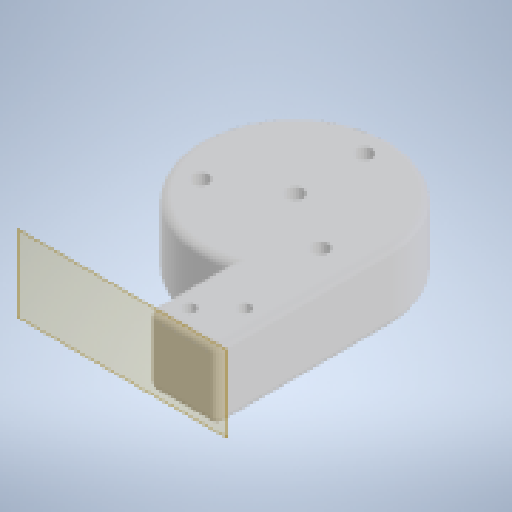
# Autodesk Inventor part: PulleytoHand
Saved by Autodesk Inventor 2024 (Build 280153000, 153)
## iProperties
Created: 2024-02-21
Part Number: PulleytoHand
Material: PC/ABS Plastic
Document SubType Name: Modeling
Designer: Irwin
Density: 0.357273 g/cm^3
Appearance: Smooth - White
Author: Irwin
Autodesk Inventor part; units mm, degrees
ref_plane "YZ Plane" through (0, 0, 0) normal (1, 0, 0) x (0, 1, 0)
ref_plane "XZ Plane" through (0, 0, 0) normal (0, 1, 0) x (-1, 0, 0)
sketch "Sketch1" plane through (0, 0, 0) normal (0, 1, 0) x (-1, 0, 0)
  circle A0 centre (0, 0) radius 27.5
  dimension "d0" = 55
  constraints: 1 centre point, 1 coincident
  measures "d0" diameter of A0
extrude "Extrusion1" add sketch "Sketch1" along normal blind 20
ref_plane "Work Plane1" through (0, 0, 50) normal (0, 0, 1) x (1, 0, 0)
sketch "Sketch5" plane through (0, 0, 50) normal (0, 0, 1) x (1, 0, 0)
  line L0 (27.5, 20) -> (-27.5, 20) projected
  line L1 (27.5, 0) -> (27.5, 20) projected
  line L2 (27.5, 0) -> (-27.5, 0) projected
  line L3 (27.5, 20) -> (7.5, 20)
  line L4 (7.5, 20) -> (7.5, 0)
  line L5 (7.5, 0) -> (27.5, 0)
  line L6 (27.5, 0) -> (27.5, 20)
  point P0 (0, 0)
  dimension "d24" = 20
  constraints: 8 end point, 2 parallel, 1 horizontal, 1 perpendicular, 1 point on line
  measures "d24" distance of L5.end L4.end
extrude "Extrusion4" add sketch "Sketch5" against normal through all
sketch "Sketch3" plane through (0, 20, 0) normal (0, 1, 0) x (1, 0, 0)
  circle A0 centre (0, 0) radius 20 construction
  point P0 (0, 20)
  point P1 (-17.3205, -10)
  point P2 (17.3205, -10)
  dimension "d6" = 20
  dimension "d7" = 40
  dimension "d10" = 360
  constraints: 1 centre point, 1 coincident, 1 vertical alignment, 4 other
  measures "d6" distance of point (0, 0) point (0, 20)
  measures "d7" diameter of A0
hole "Hole1" at (0, 20, -20) at (-17.3205, 20, 10) at (17.3205, 20, 10) direction (0, -1, 0) diameter 4.8 end through all clearance for "Flat Head Machine Screw" size "M4" standard "Ansi Metric M Profile"
fillet "Fillet2" radius 2 10 edges at (27.5, 20, 25) (-21.9374, 20, -16.5831) (-21.9374, 0, -16.5831) (27.5, 0, 25) (7.5, 20, 38.2288) (7.5, 0, 38.2288) (17.5, 20, 50) (7.5, 10, 50) (17.5, 0, 50) (27.5, 10, 50)
sketch "Sketch6" plane through (0, 20, 0) normal (0, 1, 0) x (1, 0, 0)
  line L0 (38.5, -50) -> (-38.5, -50) projected
  line L1 (27.5, -48) -> (27.5, 0) projected
  point P0 (0, 0)
  point P1 (13.5, -44)
  point P2 (13.5, -36)
  point P3 (21.5, -36)
  point P4 (21.5, -44)
  dimension "d28" = 6
  dimension "d29" = 8
  dimension "d30" = 8
  dimension "d31" = 6
  constraints: 2 horizontal alignment, 2 vertical alignment
  measures "d28" distance from line of L0 point (13.5, -44)
  measures "d29" distance of point (21.5, -44) point (21.5, -36)
  measures "d30" distance of point (13.5, -36) point (21.5, -36)
  measures "d31" distance from line of L1 point (21.5, -36)
hole "Hole2" at (13.5, 20, 44) at (21.5, 20, 36) direction (0, -1, 0) diameter 3.6 end through all clearance for "Flat Head Machine Screw" size "M3" standard "Ansi Metric M Profile"
sketch "Sketch2" plane through (0, 0, 0) normal (0, -1, 0) x (1, 0, 0)
  circle A0 centre (0, 0) radius 16
  dimension "d3" = 32
  constraints: 1 centre point, 1 coincident
  measures "d3" diameter of A0
extrude "Extrusion2" cut sketch "Sketch2" against normal blind 8
sketch "Sketch7" plane through (0, 20, 0) normal (0, 1, 0) x (1, 0, 0)
  circle A0 centre (0, 0) radius 2.5
  dimension "d39" = 5
  constraints: 1 centre point, 1 coincident
  measures "d39" diameter of A0
extrude "Extrusion5" cut sketch "Sketch7" against normal through all
body "Solid1"
